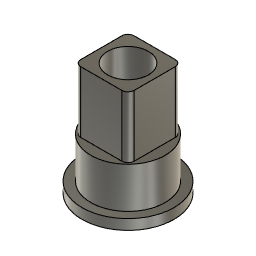
WindingSteam v2 (Autodesk Fusion 360 design; units mm, degrees)
Autodesk Fusion 360 part; units mm, degrees
sketch "bottom" plane through (0, 0, 0) normal (0, 0, 1) x (1, 0, 0)
  circle A0 centre (0, 0) radius 2.25
  circle A1 centre (0, 0) radius 5
  line L0 (5.04, 6.54) -> (-5.04, 6.54)
  line L1 (-6.54, 5.04) -> (-6.54, -5.04)
  line L2 (-5.04, -6.54) -> (5.04, -6.54)
  line L3 (6.54, -5.04) -> (6.54, 5.04)
  line L4 (6.54, 6.54) -> (-6.54, -6.54) construction
  line L5 (-6.54, 6.54) -> (6.54, -6.54) construction
  arc A2 (-5.04, 6.54) -> (-6.54, 5.04) centre (-5.04, 5.04) ccw
  arc A3 (6.54, 5.04) -> (5.04, 6.54) centre (5.04, 5.04) ccw
  arc A4 (5.04, -6.54) -> (6.54, -5.04) centre (5.04, -5.04) ccw
  arc A5 (-6.54, -5.04) -> (-5.04, -6.54) centre (-5.04, -5.04) ccw
  circle A6 centre (0, 0) radius 9.1
  circle A7 centre (0, 0) radius 11.25
  dimension "d1" = 4.5
  dimension "d2" = 10
  dimension "d3" = 13.08
  dimension "d4" = 13.08
  dimension "d5" = 1.5
  dimension "d6" = 18.2
  dimension "d7" = 22.5
  constraint coincident A0.centre A1.centre
  constraint concentric A0 A1
  constraint horizontal L0
  constraint perpendicular L0 L1
  constraint parallel L0 L2
  constraint parallel L1 L3
  constraint coincident L4 A0.centre
  constraint coincident L5 A0.centre
  constraint coincident L5.start L0
  constraint coincident L5.start L1
  constraint tangent L0 A2
  constraint tangent L1 A2
  constraint coincident L4.start L0
  constraint coincident L4.start L3
  constraint tangent L0 A3
  constraint tangent L3 A3
  constraint equal A2 A3
  constraint coincident L5.end L3
  constraint coincident L5.end L2
  constraint tangent L3 A4
  constraint tangent L2 A4
  constraint equal A2 A4
  constraint coincident L4.end L2
  constraint coincident L4.end L1
  constraint tangent L2 A5
  constraint tangent L1 A5
  constraint equal A2 A5
  constraint concentric A1 A6
  constraint concentric A6 A7
  measures "d1" diameter of A0
  measures "d2" diameter of A1
  measures "d3" distance of L4.end L5.end
  measures "d4" distance of L5.start L4.end
  measures "d5" radius of A2
  measures "d6" diameter of A6
  measures "d7" diameter of A7
extrude "Extrude1" add sketch "bottom" along normal blind 27.5 and the other way blind -7.5 contours L0 L1 L2 L3 A2 A3 A4 A5
extrude "Extrude2" add sketch "bottom" along normal blind 12.5 and the other way blind -7.5 contours A1
extrude "Extrude3" add sketch "bottom" along normal blind 12.5 contours A6
extrude "Extrude4" add sketch "bottom" along normal blind 2.5 contours A7
equation "d12 = 5.00 mm + 7.50 mm"
named bodies: "WindingSteam"
